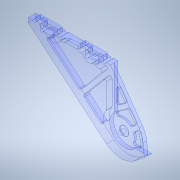
# Autodesk Inventor part: 後ろウィング固定フレームver2(ミラー)反対側
Saved by Autodesk Inventor 2020.2 (Build 242310000, 310)
## iProperties
Created: 2020-05-07
Part Number: 後ろウィング固定フレームver2(ミラー)反対側
Material: ポリカーボネート、クリア
Document SubType Name: Modeling
Designer: mozar
Density: 1.2 g/cm^3
Appearance: ポリカーボネート - クリア
Mass: 7.61117 g
Surface Area: 65.4566 cm^2
Volume: 6.34264 cm^3
Author: mozar
Autodesk Inventor part; units mm, degrees
(part 1 of 2)
ref_plane "YZ Plane" through (0, 0, 0) normal (1, 0, 0) x (0, 1, 0)
ref_plane "XZ Plane" through (0, 0, 0) normal (0, 1, 0) x (-1, 0, 0)
ref_plane "XY Plane" through (0, 0, 0) normal (0, 0, 1) x (1, 0, 0)
sketch "スケッチ1" plane through (0, 0, 0) normal (0, 0, 1) x (1, 0, 0)
  line L0 (-101.5, 47.999998) -> (108.5, 47.999998)
  circle A0 centre (111.885049, -39.000002) radius 4
  circle A1 centre (191.876682, -37.842982) radius 4
  circle A2 centre (111.885049, -39.000002) radius 7
  circle A3 centre (191.876682, -37.842982) radius 7
  line L1 (191.876682, -37.842982) -> (111.885049, -39.000002) construction
  line L2 (191.775442, -30.843714) -> (111.78381, -32.000734)
  line L3 (111.986288, -45.99927) -> (191.977921, -44.84225)
  arc A4 (191.977921, -44.84225) -> (191.775442, -30.843714) centre (191.876682, -37.842982) ccw
  arc A5 (111.78381, -32.000734) -> (111.986288, -45.99927) centre (111.885049, -39.000002) ccw
  line L4 (193.542302, -31.044032) -> (241.704818, -42.842982)
  circle A6 centre (234.566446, -71.981335) radius 30
  line L5 (262.587356, -82.697145) -> (213.725294, -50.402494)
  line L6 (213.725294, -50.402494) -> (190.211062, -44.641931)
  line L7 (264.566446, -121.542906) -> (264.566446, -63.2267)
  line L8 (111.885049, -39.000002) -> (111.885049, 40.999998) construction
  line L9 (118.885049, -39.000002) -> (118.885049, 40.999998)
  line L10 (104.885049, 40.999998) -> (104.885049, -39.000002)
  arc A7 (104.885049, -39.000002) -> (118.885049, -39.000002) centre (111.885049, -39.000002) ccw
  arc A8 (118.885049, 40.999998) -> (104.885049, 40.999998) centre (111.885049, 40.999998) ccw
  circle A9 centre (58.238326, 51.481995) radius 30
  line L11 (113.558078, 34.202868) -> (65.408448, 22.351438)
  line L12 (28.441083, 47.999998) -> (86.70408, 42.010942)
  line L13 (86.70408, 42.010942) -> (110.21202, 47.797128)
  circle A10 centre (113.5, -20.000002) radius 68
  line L14 (315.327237, -100.585467) -> (70.600424, 104.764712)
  line L15 (253.850074, -49.000002) -> (111.885049, -39.000002)
  arc A11 (93.592427, -27.104845) -> (135.370976, -5.924402) centre (95.060351, 21.794105) ccw
  arc A12 (135.370976, -5.924402) -> (135.847591, -3.671647) centre (132.898992, -4.224609) ccw
  arc A13 (135.847591, -3.671647) -> (83.183341, 18.55647) centre (102.157897, -9.989602) ccw
  line L16 (111.885049, -39.000002) -> (112.74718, 40.995353) construction
  line L17 (118.884642, -39.075438) -> (119.746773, 40.919916)
  line L18 (105.747586, 41.070789) -> (104.885455, -38.924565)
  arc A14 (104.885455, -38.924565) -> (118.884642, -39.075438) centre (111.885049, -39.000002) ccw
  arc A15 (119.746773, 40.919916) -> (105.747586, 41.070789) centre (112.74718, 40.995353) ccw
  line L19 (164.994898, 47.999998) -> (164.994898, 25.999998)
  line L20 (164.994898, 25.999998) -> (327.494898, -102.000002)
  circle A16 centre (116.292557, -40.000002) radius 68
  circle A17 centre (-98.885049, -0.000002) radius 67.5
  line L21 (321.363327, -8.500986) -> (-152.668056, 78.49822)
  line L22 (104.889695, -3) -> (104.889695, 0)
  line L23 (104.889695, -3) -> (64.444342, -3)
  line L24 (72.06562, 0) -> (104.889695, 0)
  circle A18 centre (83.376901, -17.5) radius 13.85
  line L25 (198.510163, -35.607602) -> (190.779082, -12.66564)
  line L26 (185.2432, -40.078361) -> (169.408182, 6.912014)
  circle A19 centre (197.837389, 16.492211) radius 30
  line L27 (190.779082, -12.66564) -> (191.876682, 45.894081)
  circle A20 centre (191.876682, -37.842982) radius 83.737063
  line L28 (191.876682, 45.894081) -> (191.876682, -37.842982)
  line L29 (96.889695, -3) -> (96.889695, -6)
  line L30 (96.889695, -6) -> (87.889695, -6)
  line L31 (87.889695, -6) -> (87.889695, -3)
  line L32 (76.444342, -3) -> (76.444342, -6)
  line L33 (76.444342, -6) -> (67.444342, -6)
  line L34 (67.444342, -6) -> (67.444342, -3)
  line L35 (99.889695, -3) -> (99.889695, 0)
  line L36 (99.889695, 0) -> (84.889695, 0)
  line L37 (84.889695, 0) -> (84.889695, -3)
  line L38 (79.444342, -3) -> (79.444342, 0)
  line L39 (79.444342, 0) -> (64.444342, 0)
  line L40 (64.444342, 0) -> (64.444342, -3)
  line L41 (64.444342, 0) -> (59.444342, 0)
  line L42 (59.444342, 0) -> (59.444342, -3)
  line L43 (59.444342, -3) -> (64.444342, -3)
  line L44 (59.444342, -3) -> (59.444342, -6)
  circle A21 centre (111.885049, -39.000002) radius 1.5
  circle A22 centre (111.885049, -39.000002) radius 9
  circle A23 centre (111.885049, -39.000002) radius 10
  circle A24 centre (111.885049, -39.000002) radius 15
  line L45 (121.057661, -50.868582) -> (142.927269, -50.552254)
  line L46 (121.057661, -50.868582) -> (127.651316, -45.772687)
  line L47 (127.651316, -45.772687) -> (126.808053, -37.482129)
  line L48 (124.15135, -30.366471) -> (104.889695, -3)
  line L49 (101.060181, -49.383751) -> (59.444342, -6)
  circle A25 centre (95.889695, -6) radius 1
  circle A26 centre (88.889695, -6) radius 1
  circle A27 centre (95.889695, -3) radius 1
  circle A28 centre (88.889695, -3) radius 1
  circle A29 centre (100.889695, -3) radius 1
  circle A30 centre (83.889695, -3) radius 1
  circle A31 centre (80.444342, -3) radius 1
  circle A32 centre (75.444342, -6) radius 1
  circle A33 centre (68.444342, -6) radius 1
  circle A34 centre (75.444342, -3) radius 1
  circle A35 centre (68.444342, -3) radius 1
  circle A36 centre (63.444342, -3) radius 1
  point P0 (0, 0)
  point P1 (151.880865, -38.421492)
  point P2 (111.885049, 0.999998)
  point P3 (105.885049, -0.000002)
  point P4 (105.885049, -0.000002)
  point P5 (23.732778, -42.728965)
  point P6 (112.316114, 0.997675)
  point P7 (99.889695, -1.5)
  point P8 (76.444342, -4.5)
  point P9 (74.444342, -6)
  point P10 (69.444342, -6)
  point P11 (69.444342, -3)
  point P12 (74.444342, -3)
  point P13 (82.889695, -3)
  point P14 (81.444342, -3)
  point P15 (62.444342, -3)
  point P16 (101.889695, -3)
  point P17 (89.889695, -3)
  point P18 (94.889695, -3)
  point P19 (94.889695, -6)
  point P20 (89.889695, -6)
  point P21 (118.961603, -31.934425)
  point P22 (118.924491, -31.897449)
  point P23 (118.962007, -31.896907)
  point P24 (119.12697, -45.895985)
  point P25 (104.885049, -3)
  point P26 (104.885049, -31.858573)
  dimension "d27" = 167.47413
  dimension "d0" = 8
  dimension "d1" = 8
  dimension "d2" = 3
  dimension "d3" = 3
  dimension "d4" = 80
  dimension "d5" = 14
  dimension "d6" = 14
  dimension "d7" = 60
  dimension "d8" = 14
  dimension "d9" = 60
  dimension "d10" = 14
  dimension "d11" = 6
  dimension "d12" = 40
  dimension "d13" = 13.271
  dimension "d14" = 14
  dimension "d15" = 10
  dimension "d16" = 5
  dimension "d17" = 22
  dimension "d18" = 150
  dimension "d19" = 162.5
  dimension "d20" = 0
  dimension "d21" = 136
  dimension "d22" = 136
  dimension "d23" = 135
  dimension "d24" = 38.2272
  dimension "d25" = 25
  dimension "d26" = 60
  dimension "d28" = 5
  dimension "d29" = 3
  dimension "d30" = 5
  dimension "d31" = 3
  dimension "d32" = 3
  dimension "d33" = 5
  dimension "d34" = 1
  dimension "d35" = 5
  dimension "d36" = 5
  dimension "d37" = 2
  dimension "d38" = 2
  dimension "d39" = 2
  dimension "d40" = 2
  dimension "d41" = 2
  dimension "d42" = 2
  dimension "d43" = 2
  dimension "d44" = 2
  dimension "d45" = 2
  dimension "d46" = 2
  dimension "d47" = 2
  dimension "d48" = 2
  constraints: 104 end point, 46 tangent, 37 point on circle, 36 centre point, 14 vertical, 8 point on line, 7 equal length, 7 horizontal, 5 coincident, 5 midpoint, 5 parallel, 1 concentric, 1 perpendicular, 1 vertical alignment, 25 other
  measures "d0" diameter of A0
  measures "d1" diameter of A1
  measures "d2" radial gap between concentric circles of A0 A2
  measures "d3" radial gap between concentric circles of A1 A3
  measures "d4" distance of L1.start L1.end
  measures "d5" diameter of A5
  measures "d6" distance from line of L4 L5.end
  measures "d7" diameter of A6
  measures "d8" diameter of A8
  measures "d9" diameter of A9
  measures "d10" distance from line of L11 L12.end
  measures "d11" horizontal distance of L1.end point (105.885, 0)
  measures "d12" angle of L14 L0
  measures "d14" diameter of A15
  measures "d15" vertical distance of L15.start L1.end
  measures "d16" vertical distance of L1.start L4.end
  measures "d17" distance of L19.start L19.end
  measures "d18" vertical distance of L19.start L20.end
  measures "d19" distance from line of L19 L20.end
  measures "d20" distance from line of L19.start L0
  measures "d21" diameter of A10
  measures "d22" diameter of A16
  measures "d23" diameter of A17
  measures "d24" angle of L0 L20
  measures "d25" distance from line of L5.start L20
  measures "d26" diameter of A19
  measures "d28" distance between parallel lines of L35 L22
  measures "d29" distance of L41.end L42.end
  measures "d30" distance of L42.end L40.end
  measures "d31" distance of L42.end L44.end
  measures "d32" diameter of A21
  measures "d33" radial gap between concentric circles of A0 A22
  measures "d34" radial gap between concentric circles of A22 A23
  measures "d35" radial gap between concentric circles of A23 A24
  measures "d36" distance between parallel lines of L3 L45
  measures "d37" diameter of A25
  measures "d38" diameter of A26
  measures "d39" diameter of A27
  measures "d40" diameter of A28
  measures "d41" diameter of A29
  measures "d42" diameter of A30
  measures "d43" diameter of A31
  measures "d44" diameter of A32
  measures "d45" diameter of A33
  measures "d46" diameter of A34
  measures "d47" diameter of A35
  measures "d48" diameter of A36
extrude "押し出し1" add sketch "スケッチ1" against normal blind 5 contours A24 A11 L10 A23 A20 | A20 A23 L3 A24 | L43 A36 L23 L34 A33 L33 A32 A18 L49 L44 | L46 A24 L3 | L3 A24 L15 L47 | A23 L10 A22 A20 | A20 A22 L3 A23 | L49 A18 L30 A25 L29 L23 A29 L10 A24 | L39 L24 L38 L23 A34 A35 L40 | L3 A23 L15 A24 | L15 A24 L47 | A22 L10 A2 A20 | A20 A2 L3 A22 | A23 L18 A22 L10 | L10 A11 L18 A23 | L3 A22 L15 A23 | A24 L10 A11 | L49 A18 A32 L32 A31 A30 L31 A26 L30 | L15 A23 L17 L2 A24 | L2 L17 A24 | A20 A0 L15 A2 | A2 A20 A0 | A22 L18 L10 | L3 A2 L15 A22 | L10 A24 L18 A11 | A23 A20 A22 L18 | L18 A11 A20 A23 | L15 A22 L17 A23 | L10 L23 L48 L18 A24 | L35 L23 A27 A28 L37 L24 | L48 A20 A24 L18 | L17 A23 L2 | L2 A23 L9 A24 L17 | A24 L17 L48 | A20 A0 | A0 A20 | L18 A22 A20 A2 | L15 A2 L17 A22 | L18 A24 A20 A11 | A23 L9 L2 A22 A20 | A20 A11 A24 L9 A23 | A31 A18 L32 L23 | L48 A11 A24 A20 | A23 L17 A22 L9 L2 | L2 L9 A23 | A24 L9 L48 L17 | L15 A0 A20 A2 | A20 A22 L2 A2 | A20 A24 A11 | A18 A30 L23 L31 | L23 A30 A18 A31 | L48 L9 A24 A11 | L9 A22 L2 | L17 L9 A22 | L2 A22 L9 A2
extrude "押し出し2" cut sketch "スケッチ1" against normal blind 2.55 contours L3 A24 L15 L47 | A23 L10 A22 A20 | A20 A22 L3 A23 | L3 A23 L15 A24 | L15 A24 L47 | A22 L10 A2 A20 | A20 A2 L3 A22 | A23 L18 A22 L10 | L10 A11 L18 A23 | L3 A22 L15 A23 | L15 A23 L17 L2 A24 | L2 L17 A24 | A20 A0 L15 A2 | A2 A20 A0 | A22 L18 L10 | L3 A2 L15 A22 | L10 A24 L18 A11 | A23 A20 A22 L18 | L18 A11 A20 A23 | L15 A22 L17 A23 | L10 L23 L48 L18 A24 | L48 A20 A24 L18 | L17 A23 L2 | L2 A23 L9 A24 L17 | A24 L17 L48 | A20 A0 | A0 A20 | L18 A22 A20 A2 | L15 A2 L17 A22 | L18 A24 A20 A11 | A23 L9 L2 A22 A20 | A20 A11 A24 L9 A23 | L48 A11 A24 A20 | A23 L17 A22 L9 L2 | L2 L9 A23 | A24 L9 L48 L17 | L15 A0 A20 A2 | A20 A22 L2 A2 | A20 A24 A11 | L48 L9 A24 A11 | L9 A22 L2 | L17 L9 A22 | L2 A22 L9 A2 | A21
sketch "スケッチ2" plane through (0, 0, 0) normal (0, 0, 1) x (1, 0, 0)
  line L0 (87.889695, -6) -> (87.889695, -3)
  arc A0 (89.889695, -3) -> (87.889695, -3) centre (88.889695, -3) ccw
  line L1 (89.889695, -3) -> (94.889695, -3)
  arc A1 (96.889695, -3) -> (94.889695, -3) centre (95.889695, -3) ccw
  line L2 (96.889695, -3) -> (96.889695, -6)
  arc A2 (94.889695, -6) -> (96.889695, -6) centre (95.889695, -6) ccw
  line L3 (94.889695, -6) -> (89.889695, -6)
  arc A3 (87.889695, -6) -> (89.889695, -6) centre (88.889695, -6) ccw
  arc A4 (67.444342, -6) -> (69.444342, -6) centre (68.444342, -6) ccw
  line L4 (67.444342, -6) -> (67.444342, -3)
  arc A5 (69.444342, -3) -> (67.444342, -3) centre (68.444342, -3) ccw
  line L5 (69.444342, -3) -> (74.444342, -3)
  arc A6 (76.444342, -3) -> (74.444342, -3) centre (75.444342, -3) ccw
  line L6 (76.444342, -3) -> (76.444342, -6)
  arc A7 (74.444342, -6) -> (76.444342, -6) centre (75.444342, -6) ccw
  line L7 (74.444342, -6) -> (69.444342, -6)
  line L8 (127.651316, -45.772687) -> (119.12697, -45.895985)
  arc A8 (104.885049, -31.858573) -> (119.12697, -45.895985) centre (111.885049, -39.000002) ccw
  line L9 (104.885049, -31.858573) -> (104.885049, -3)
  line L10 (104.885049, -3) -> (101.889695, -3)
  arc A9 (99.889695, -3) -> (101.889695, -3) centre (100.889695, -3) ccw
  line L11 (99.889695, -3) -> (99.889695, 0)
  line L12 (99.889695, 0) -> (84.889695, 0)
  line L13 (84.889695, 0) -> (84.889695, -3)
  arc A10 (82.889695, -3) -> (84.889695, -3) centre (83.889695, -3) ccw
  line L14 (82.889695, -3) -> (81.444342, -3)
  arc A11 (79.444342, -3) -> (81.444342, -3) centre (80.444342, -3) ccw
  line L15 (79.444342, -3) -> (79.444342, 0)
  line L16 (79.444342, 0) -> (64.444342, 0)
  line L17 (64.444342, 0) -> (64.444342, -3)
  arc A12 (62.444342, -3) -> (64.444342, -3) centre (63.444342, -3) ccw
  line L18 (62.444342, -3) -> (59.444342, -3)
  line L19 (59.444342, -3) -> (59.444342, -6)
  line L20 (59.444342, -6) -> (101.060181, -49.383751)
  arc A13 (101.060181, -49.383751) -> (121.057661, -50.868582) centre (111.885049, -39.000002) ccw
  line L21 (121.057661, -50.868582) -> (127.651316, -45.772687)
  circle A14 centre (111.885049, -39.000002) radius 1.5
  circle A15 centre (111.885049, -39.000002) radius 3
  point P0 (0, 0)
  dimension "d53" = 6
  constraints: 1 centre point, 1 coincident
  measures "d53" diameter of A15
extrude "押し出し3" cut sketch "スケッチ2" against normal blind 3 contours A15
sketch "スケッチ3" plane through (0, 0, 0) normal (0, 0, 1) x (1, 0, 0)
  line L0 (87.889695, -6) -> (87.889695, -3)
  arc A0 (89.889695, -3) -> (87.889695, -3) centre (88.889695, -3) ccw
  line L1 (89.889695, -3) -> (94.889695, -3)
  arc A1 (96.889695, -3) -> (94.889695, -3) centre (95.889695, -3) ccw
  line L2 (96.889695, -3) -> (96.889695, -6)
  arc A2 (94.889695, -6) -> (96.889695, -6) centre (95.889695, -6) ccw
  line L3 (94.889695, -6) -> (89.889695, -6)
  arc A3 (87.889695, -6) -> (89.889695, -6) centre (88.889695, -6) ccw
  arc A4 (67.444342, -6) -> (69.444342, -6) centre (68.444342, -6) ccw
  line L4 (67.444342, -6) -> (67.444342, -3)
  arc A5 (69.444342, -3) -> (67.444342, -3) centre (68.444342, -3) ccw
  line L5 (69.444342, -3) -> (74.444342, -3)
  arc A6 (76.444342, -3) -> (74.444342, -3) centre (75.444342, -3) ccw
  line L6 (76.444342, -3) -> (76.444342, -6)
  arc A7 (74.444342, -6) -> (76.444342, -6) centre (75.444342, -6) ccw
  line L7 (74.444342, -6) -> (69.444342, -6)
  line L8 (127.651316, -45.772687) -> (119.12697, -45.895985)
  arc A8 (104.885049, -31.858573) -> (119.12697, -45.895985) centre (111.885049, -39.000002) ccw
  line L9 (104.885049, -31.858573) -> (104.885049, -3)
  line L10 (104.885049, -3) -> (101.889695, -3)
  arc A9 (99.889695, -3) -> (101.889695, -3) centre (100.889695, -3) ccw
  line L11 (99.889695, -3) -> (99.889695, 0)
  line L12 (99.889695, 0) -> (84.889695, 0)
  line L13 (84.889695, 0) -> (84.889695, -3)
  arc A10 (82.889695, -3) -> (84.889695, -3) centre (83.889695, -3) ccw
  line L14 (82.889695, -3) -> (81.444342, -3)
  arc A11 (79.444342, -3) -> (81.444342, -3) centre (80.444342, -3) ccw
  line L15 (79.444342, -3) -> (79.444342, 0)
  line L16 (79.444342, 0) -> (64.444342, 0)
  line L17 (64.444342, 0) -> (64.444342, -3)
  arc A12 (62.444342, -3) -> (64.444342, -3) centre (63.444342, -3) ccw
  line L18 (62.444342, -3) -> (59.444342, -3)
  line L19 (59.444342, -3) -> (59.444342, -6)
  line L20 (59.444342, -6) -> (101.060181, -49.383751)
  arc A13 (101.060181, -49.383751) -> (121.057661, -50.868582) centre (111.885049, -39.000002) ccw
  line L21 (121.057661, -50.868582) -> (127.651316, -45.772687)
  line L22 (99.889695, 0) -> (99.889695, -3)
  line L23 (99.889695, 0) -> (64.444342, 0)
  line L24 (64.444342, 0) -> (64.444342, -3)
  line L25 (64.444342, -3) -> (99.889695, -3)
  line L26 (99.889695, -3) -> (99.889695, 0)
  point P0 (0, 0)
  constraints: 8 end point, 2 parallel, 1 horizontal, 1 perpendicular
extrude "押し出し4" cut sketch "スケッチ3" against normal blind 2 contours L25 L13 L12 L11 A1 L1 A0 | A0 L25 | L25 L14 L15 L23 L13 | A1 L25 | L15 L25 A6 L5 A5 L17 L16 | L25 A6 | A5 L25
sketch "スケッチ4" plane through (0, 0, -5) normal (0, 0, -1) x (-1, 0, 0)
  circle A0 centre (-111.885049, -39.000002) radius 3
  line L0 (-104.885049, -3) -> (-104.889695, -3)
  line L1 (-104.885049, -31.858573) -> (-104.885049, -3)
  arc A1 (-119.12697, -45.895985) -> (-104.885049, -31.858573) centre (-111.885049, -39.000002) ccw
  line L2 (-127.651316, -45.772687) -> (-119.12697, -45.895985)
  line L3 (-126.808053, -37.482129) -> (-127.651316, -45.772687)
  arc A2 (-124.15135, -30.366471) -> (-126.808053, -37.482129) centre (-111.885049, -39.000002) ccw
  line L4 (-104.889695, -3) -> (-124.15135, -30.366471)
  circle A3 centre (-111.885049, -39.000002) radius 1.5
  point P0 (0, 0)
sketch "スケッチ5" plane through (0, 0, 0) normal (0, 0, 1) x (1, 0, 0)
  circle A0 centre (111.885049, -39.000002) radius 3
  line L0 (104.885049, -3) -> (104.889695, -3)
  line L1 (104.885049, -31.858573) -> (104.885049, -3)
  arc A1 (104.885049, -31.858573) -> (119.12697, -45.895985) centre (111.885049, -39.000002) ccw
  line L2 (127.651316, -45.772687) -> (119.12697, -45.895985)
  line L3 (126.808053, -37.482129) -> (127.651316, -45.772687)
  arc A2 (126.808053, -37.482129) -> (124.15135, -30.366471) centre (111.885049, -39.000002) ccw
  line L4 (104.889695, -3) -> (124.15135, -30.366471)
  circle A3 centre (111.885049, -39.000002) radius 1.5
  point P0 (0, 0)
extrude "押し出し5" add sketch "スケッチ5" against normal blind 3 contours A0 | L0 L4 A2 L3 L2 A1 L1
extrude "押し出し6" cut sketch "スケッチ4" against normal blind 3 contours A0
extrude "押し出し7" cut sketch "スケッチ4" against normal blind 2.55 contours L1 A1 L2 L3 A2 L4 L0
sketch "スケッチ6" plane through (0, 0, -5) normal (0, 0, -1) x (-1, 0, 0)
  line L0 (-79.444342, 0) -> (-79.444342, -3)
  line L1 (-64.444342, 0) -> (-79.444342, 0)
  line L2 (-64.444342, -3) -> (-64.444342, 0)
  line L3 (-67.444342, -3) -> (-64.444342, -3)
  arc A0 (-67.444342, -3) -> (-69.444342, -3) centre (-68.444342, -3) ccw
  line L4 (-74.444342, -3) -> (-69.444342, -3)
  arc A1 (-74.444342, -3) -> (-76.444342, -3) centre (-75.444342, -3) ccw
  line L5 (-79.444342, -3) -> (-76.444342, -3)
  arc A2 (-94.889695, -3) -> (-96.889695, -3) centre (-95.889695, -3) ccw
  line L6 (-99.889695, -3) -> (-96.889695, -3)
  line L7 (-99.889695, 0) -> (-99.889695, -3)
  line L8 (-84.889695, 0) -> (-99.889695, 0)
  line L9 (-84.889695, -3) -> (-84.889695, 0)
  line L10 (-87.889695, -3) -> (-84.889695, -3)
  arc A3 (-87.889695, -3) -> (-89.889695, -3) centre (-88.889695, -3) ccw
  line L11 (-94.889695, -3) -> (-89.889695, -3)
  point P0 (0, 0)
sketch "スケッチ7" plane through (0, 0, 0) normal (0, 0, 1) x (1, 0, 0)
  arc A0 (96.889695, -3) -> (94.889695, -3) centre (95.889695, -3) ccw
  line L0 (99.889695, -3) -> (96.889695, -3)
  line L1 (99.889695, 0) -> (99.889695, -3)
  line L2 (84.889695, 0) -> (99.889695, 0)
  line L3 (84.889695, -3) -> (84.889695, 0)
  line L4 (87.889695, -3) -> (84.889695, -3)
  arc A1 (89.889695, -3) -> (87.889695, -3) centre (88.889695, -3) ccw
  line L5 (94.889695, -3) -> (89.889695, -3)
  line L6 (79.444342, 0) -> (79.444342, -3)
  line L7 (64.444342, 0) -> (79.444342, 0)
  line L8 (64.444342, -3) -> (64.444342, 0)
  line L9 (67.444342, -3) -> (64.444342, -3)
  arc A2 (69.444342, -3) -> (67.444342, -3) centre (68.444342, -3) ccw
  line L10 (74.444342, -3) -> (69.444342, -3)
  arc A3 (76.444342, -3) -> (74.444342, -3) centre (75.444342, -3) ccw
  line L11 (79.444342, -3) -> (76.444342, -3)
  point P0 (0, 0)
extrude "押し出し8" add sketch "スケッチ7" against normal blind 5
extrude "押し出し9" cut sketch "スケッチ6" against normal blind 2
sketch "スケッチ8" plane through (0, 0, -5) normal (0, 0, -1) x (-1, 0, 0)
  line L0 (-84.889695, -3) -> (-87.889695, -3)
  line L1 (-87.889695, -3) -> (-87.889695, -6)
  arc A0 (-89.889695, -6) -> (-87.889695, -6) centre (-88.889695, -6) ccw
  line L2 (-89.889695, -6) -> (-94.889695, -6)
  arc A1 (-96.889695, -6) -> (-94.889695, -6) centre (-95.889695, -6) ccw
  line L3 (-96.889695, -6) -> (-96.889695, -3)
  line L4 (-96.889695, -3) -> (-99.889695, -3)
  arc A2 (-101.889695, -3) -> (-99.889695, -3) centre (-100.889695, -3) ccw
  line L5 (-101.889695, -3) -> (-104.885049, -3)
  line L6 (-104.885049, -3) -> (-104.885049, -31.858573)
  arc A3 (-119.12697, -45.895985) -> (-104.885049, -31.858573) centre (-111.885049, -39.000002) ccw
  line L7 (-119.12697, -45.895985) -> (-127.651316, -45.772687)
  line L8 (-127.651316, -45.772687) -> (-121.057661, -50.868582)
  arc A4 (-121.057661, -50.868582) -> (-101.060181, -49.383751) centre (-111.885049, -39.000002) ccw
  line L9 (-101.060181, -49.383751) -> (-59.444342, -6)
  line L10 (-59.444342, -6) -> (-59.444342, -3)
  line L11 (-59.444342, -3) -> (-62.444342, -3)
  arc A5 (-64.444342, -3) -> (-62.444342, -3) centre (-63.444342, -3) ccw
  line L12 (-64.444342, -3) -> (-67.444342, -3)
  line L13 (-67.444342, -3) -> (-67.444342, -6)
  arc A6 (-69.444342, -6) -> (-67.444342, -6) centre (-68.444342, -6) ccw
  line L14 (-69.444342, -6) -> (-74.444342, -6)
  arc A7 (-76.444342, -6) -> (-74.444342, -6) centre (-75.444342, -6) ccw
  line L15 (-76.444342, -6) -> (-76.444342, -3)
  line L16 (-76.444342, -3) -> (-79.444342, -3)
  arc A8 (-81.444342, -3) -> (-79.444342, -3) centre (-80.444342, -3) ccw
  line L17 (-81.444342, -3) -> (-82.889695, -3)
  arc A9 (-84.889695, -3) -> (-82.889695, -3) centre (-83.889695, -3) ccw
  line L18 (-66.444342, -6) -> (-57.444342, -6)
  line L19 (-57.444342, -6) -> (-57.444342, -3)
  line L20 (-57.444342, -3) -> (-66.444342, -3)
  line L21 (-66.444342, -3) -> (-66.444342, -6)
  line L22 (-69.444342, -6) -> (-74.444342, -6)
  line L23 (-64.444342, -3) -> (-67.444342, -3)
  circle A10 centre (-65.444342, -3) radius 1
  circle A11 centre (-65.444342, -6) radius 1
  circle A12 centre (-58.444342, -3) radius 1
  circle A13 centre (-58.444342, -6) radius 1
  line L24 (-54.444342, 0) -> (-54.444342, -6)
  line L25 (-61.090093, -9) -> (-62.79859, -9)
  line L26 (-69.444342, -6) -> (-69.444342, 0)
  line L27 (-69.444342, 0) -> (-54.444342, 0)
  circle A14 centre (-65.444342, -6) radius 4
  circle A15 centre (-58.444342, -6) radius 4
  line L28 (-64.444342, 0) -> (-64.444342, -3)
  line L29 (-79.444342, -3) -> (-79.444342, 0)
  line L30 (-69.444342, 0) -> (-54.444342, 0)
  line L31 (-54.444342, 0) -> (-54.444342, -3)
  line L32 (-54.444342, -3) -> (-69.444342, -3)
  line L33 (-69.444342, -3) -> (-69.444342, 0)
  line L34 (-54.444342, -3) -> (-49.444342, -3)
  line L35 (-49.444342, -3) -> (-49.444342, -6)
  line L36 (-49.444342, -6) -> (-54.444342, -6)
  line L37 (-54.444342, -6) -> (-54.444342, -3)
  circle A16 centre (-53.444342, -3) radius 1
  circle A17 centre (-70.444342, -3) radius 1
  line L38 (-76.444342, -3) -> (-69.444342, -3)
  line L39 (-79.444342, 0) -> (-64.444342, 0)
  line L40 (-79.444342, 0) -> (-64.444342, 0)
  line L41 (-81.444342, -3) -> (-79.444342, -3)
  point P0 (0, 0)
  point P1 (-61.944342, -3)
  point P2 (-52.444342, -3)
  point P3 (-71.444342, -3)
  point P4 (-59.444342, -6)
  point P5 (-64.444342, -6)
  dimension "d68" = 9
  dimension "d69" = 3
  dimension "d70" = 10
  dimension "d71" = 2
  dimension "d72" = 2
  dimension "d73" = 2
  dimension "d74" = 2
  dimension "d75" = 3
  dimension "d76" = 3
  dimension "d77" = 3
  dimension "d78" = 3
  dimension "d79" = 15
  dimension "d80" = 15
  dimension "d81" = 3
  dimension "d82" = 3
  dimension "d83" = 15
  dimension "d84" = 3
  dimension "d85" = 10
  dimension "d86" = 2
  dimension "d88" = 2
  constraints: 38 end point, 8 centre point, 8 parallel, 7 point on line, 7 tangent, 4 horizontal, 4 perpendicular, 4 point on circle, 2 midpoint, 1 collinear
  measures "d68" distance of L20.end L19.end
  measures "d69" distance of L19.end L18.end
  measures "d70" distance between parallel lines of L15 L21
  measures "d71" diameter of A10
  measures "d72" diameter of A11
  measures "d73" diameter of A12
  measures "d74" diameter of A13
  measures "d75" distance between parallel lines of L19 L24
  measures "d76" radial gap between concentric circles of A11 A14
  measures "d77" radial gap between concentric circles of A13 A15
  measures "d78" distance between parallel lines of L14 L25
  measures "d79" distance between parallel lines of L28 L29
  measures "d80" distance of L31.end L32.end
  measures "d81" distance of L30.end L31.end
  measures "d82" distance between parallel lines of L32 L27
  measures "d83" distance between parallel lines of L31 L33
  measures "d84" distance of L34.end L35.end
  measures "d85" distance between parallel lines of L35 L10
  measures "d86" diameter of A16
  measures "d88" diameter of A17
extrude "押し出し10" cut sketch "スケッチ8" against normal blind 10 contours L29 L39 L26 A17 L38 L16 | A17 L38 | L27 L28 A14 L32 L26 | A14 A10 L12 L32 | L28 A10 A14 | A10 L12 picked at (-70.194838, -2.619415) picked at (-65.236512, -2.450134)
extrude "押し出し11" add sketch "スケッチ8" against normal blind 5 contours L38 A17 L26 L14 A7 L15 | L27 L28 A14 L32 L26 | L32 A14 L26 | L27 L24 L32 A15 L11 L20 A14 L28 | A14 L32 L13 A6 | A6 L13 L12 L21 A11 L18 A15 A14 | A14 A10 L12 L32 | L28 A10 A14 | A14 L20 L28 | A14 A15 L9 L25 | A10 L12 | A16 L34 L35 L36 L24 | L24 A15 L32 | A14 A5 L20 | L20 A5 A14 | A10 L12 | A5 A14 A15 L18 A11 L21 A10 | L9 A15 L25 | A15 L18 A14 | A14 L18 L9 A15 | A15 L9 A13 L19 L32 | L32 A12 A15 | L11 A15 A14 A5 | A14 A15 L11 L10 L18 | L18 A15 A14 | A12 L20 | A12 L11 A15 | A12 L20 | L19 A13 L10 A12 | A13 L18 | L18 A13
extrude "押し出し12" cut sketch "スケッチ8" against normal blind 10 contours A10 L12 | A14 A5 L20 | L20 A5 A14 | A10 L12 | A5 A14 A15 L18 A11 L21 A10 | L11 A15 A14 A5 | A14 A15 L11 L10 L18 | L18 A15 A14 | A11 L18 | L18 A11 | A12 L20 | A12 L20 | L19 A13 L10 A12 | A13 L18 | L18 A13 picked at (-61.796548, -5.776456)
extrude "押し出し13" add sketch "スケッチ8" against normal blind 5 contours L41 A8
sketch "スケッチ9" plane through (0, 0, -5) normal (0, 0, -1) x (-1, 0, 0)
  line L0 (-59.444342, -6) -> (-64.444342, -6)
  arc A0 (-66.444342, -6) -> (-64.444342, -6) centre (-65.444342, -6) ccw
  line L1 (-66.444342, -6) -> (-66.444342, -3)
  arc A1 (-64.444342, -3) -> (-66.444342, -3) centre (-65.444342, -3) ccw
  line L2 (-64.444342, -3) -> (-59.444342, -3)
  arc A2 (-57.444342, -3) -> (-59.444342, -3) centre (-58.444342, -3) ccw
  line L3 (-57.444342, -3) -> (-57.444342, -6)
  arc A3 (-59.444342, -6) -> (-57.444342, -6) centre (-58.444342, -6) ccw
  line L4 (-62.32209, -9) -> (-61.090093, -9)
  arc A4 (-61.090093, -9) -> (-54.444342, -6) centre (-58.444342, -6) ccw
  line L5 (-54.444342, -6) -> (-49.444342, -6)
  line L6 (-49.444342, -6) -> (-49.444342, -3)
  line L7 (-49.444342, -3) -> (-52.444342, -3)
  arc A5 (-54.444342, -3) -> (-52.444342, -3) centre (-53.444342, -3) ccw
  line L8 (-54.444342, -3) -> (-54.444342, 0)
  line L9 (-54.444342, 0) -> (-69.444342, 0)
  line L10 (-69.444342, 0) -> (-69.444342, -3)
  arc A6 (-71.444342, -3) -> (-69.444342, -3) centre (-70.444342, -3) ccw
  line L11 (-71.444342, -3) -> (-82.889695, -3)
  arc A7 (-84.889695, -3) -> (-82.889695, -3) centre (-83.889695, -3) ccw
  line L12 (-84.889695, -3) -> (-87.889695, -3)
  line L13 (-87.889695, -3) -> (-87.889695, -6)
  arc A8 (-89.889695, -6) -> (-87.889695, -6) centre (-88.889695, -6) ccw
  line L14 (-89.889695, -6) -> (-94.889695, -6)
  arc A9 (-96.889695, -6) -> (-94.889695, -6) centre (-95.889695, -6) ccw
  line L15 (-96.889695, -6) -> (-96.889695, -3)
  line L16 (-96.889695, -3) -> (-99.889695, -3)
  arc A10 (-101.889695, -3) -> (-99.889695, -3) centre (-100.889695, -3) ccw
  line L17 (-101.889695, -3) -> (-104.885049, -3)
  line L18 (-104.885049, -3) -> (-104.885049, -31.858573)
  arc A11 (-119.12697, -45.895985) -> (-104.885049, -31.858573) centre (-111.885049, -39.000002) ccw
  line L19 (-119.12697, -45.895985) -> (-127.651316, -45.772687)
  line L20 (-127.651316, -45.772687) -> (-121.057661, -50.868582)
  arc A12 (-121.057661, -50.868582) -> (-101.060181, -49.383751) centre (-111.885049, -39.000002) ccw
  line L21 (-101.060181, -49.383751) -> (-62.32209, -9)
  circle A13 centre (-111.885049, -39.000002) radius 1.5
  line L22 (-101.060181, -49.383751) -> (-62.32209, -9)
  circle A14 centre (-111.885049, -39.000002) radius 15
  line L23 (-54.444342, -6) -> (-49.444342, -6)
  arc A15 (-121.057661, -50.868582) -> (-101.060181, -49.383751) centre (-111.885049, -39.000002) ccw
  line L24 (-102.219392, -50.47062) -> (-49.444342, -6)
  point P0 (0, 0)
  constraints: 2 end point, 1 coincident, 1 point on circle, 4 other
extrude "押し出し14" add sketch "スケッチ9" against normal blind 5 contours L4 A4 L5 L24 A12 L21
extrude "押し出し15" cut sketch "スケッチ8" against normal blind 2 contours L27 L28 A14 L32 L26 | L27 L24 L32 A15 L11 L20 A14 L28 | A14 A10 L12 L32 | L28 A10 A14 | A14 L20 L28 | A10 L12 | L32 A12 A15 | A12 L20 | A12 L11 A15 picked at (-65.236512, -2.450134) picked at (-58.518516, -2.675024)
sketch "スケッチ10" plane through (0, 0, 0) normal (0, 0, 1) x (1, 0, 0)
  circle A0 centre (111.885049, -39.000002) radius 1.5
  circle A1 centre (61.312972, -56.131867) radius 13.85
  circle A2 centre (49.826136, -69.334238) radius 1.5
  circle A3 centre (49.826136, -69.334238) radius 3
  circle A4 centre (44.533686, -75.985551) radius 4
  circle A5 centre (61.312972, -56.131867) radius 14.5
  circle A6 centre (49.826136, -69.334238) radius 4
  circle A7 centre (44.533686, -75.985551) radius 7
  circle A8 centre (29.900285, -80.42716) radius 2
  circle A9 centre (29.900285, -80.42716) radius 8
  circle A10 centre (31.840112, -37) radius 7.5
  circle A11 centre (31.840112, -37) radius 34
  point P0 (0, 0)
  dimension "d101" = 6
  dimension "d102" = 8
  dimension "d103" = 29
  dimension "d104" = 1
  dimension "d105" = 3
  dimension "d106" = 16
  dimension "d107" = 68
  constraints: 12 centre point, 4 coincident, 2 tangent, 4 other
  measures "d101" diameter of A3
  measures "d102" diameter of A4
  measures "d103" diameter of A5
  measures "d104" radial gap between concentric circles of A3 A6
  measures "d105" radial gap between concentric circles of A4 A7
  measures "d106" diameter of A9
  measures "d107" diameter of A11
sketch "スケッチ11" plane through (0, 0, 0) normal (0, 0, 1) x (1, 0, 0)
  circle A0 centre (111.885049, -39.000002) radius 1.5
  circle A1 centre (61.312972, -56.131867) radius 13.85
  circle A2 centre (49.826136, -69.334238) radius 1.5
  circle A3 centre (49.826136, -69.334238) radius 3
  circle A4 centre (55.301358, -75.167071) radius 4
  circle A5 centre (61.312972, -56.131867) radius 14.5
  circle A6 centre (49.826136, -69.334238) radius 4
  circle A7 centre (55.301358, -75.167071) radius 7
  circle A8 centre (29.900285, -80.42716) radius 2
  circle A9 centre (29.900285, -80.42716) radius 8
  circle A10 centre (31.840112, -37) radius 7.5
  circle A11 centre (31.840112, -37) radius 34
  line L0 (47.462972, -56.050002) -> (47.462972, -31.350002)
  line L1 (49.444342, -3) -> (49.444342, -6)
  line L2 (49.444342, -6) -> (49.444342, -63.831309)
  line L3 (54.444342, -63.831309) -> (54.444342, -6)
  line L4 (54.444342, -6) -> (54.444342, -3)
  line L5 (51.301358, -31.350002) -> (51.301358, -56.050002)
  line L6 (51.301358, -56.050002) -> (51.301358, -80.750002)
  line L7 (51.301358, -80.750002) -> (-20.894321, -80.750002)
  point P0 (0, 0)
  dimension "d108" = 6
  dimension "d109" = 8
  dimension "d110" = 29
  dimension "d111" = 1
  dimension "d112" = 3
  dimension "d113" = 16
  dimension "d114" = 68
  dimension "d115" = 5
  constraints: 16 end point, 12 centre point, 5 vertical, 4 coincident, 3 collinear, 2 horizontal, 2 tangent, 5 other
  measures "d108" diameter of A3
  measures "d109" diameter of A4
  measures "d110" diameter of A5
  measures "d111" radial gap between concentric circles of A3 A6
  measures "d112" radial gap between concentric circles of A4 A7
  measures "d113" diameter of A9
  measures "d114" diameter of A11
  measures "d115" distance between parallel lines of L2 L3
sketch "スケッチ12" plane through (0, 0, 0) normal (0, 0, 1) x (1, 0, 0)
  circle A0 centre (111.885049, -39.000002) radius 1.5
  circle A1 centre (61.312972, -56.131867) radius 13.85
  circle A2 centre (49.826136, -69.334238) radius 1.5
  circle A3 centre (49.826136, -69.334238) radius 3
  circle A4 centre (61.312972, -56.131867) radius 14.5
  circle A5 centre (49.826136, -69.334238) radius 4
  circle A6 centre (29.900285, -80.42716) radius 2
  circle A7 centre (29.900285, -80.42716) radius 8
  circle A8 centre (31.840112, -37) radius 7.5
  circle A9 centre (31.840112, -37) radius 34
  line L0 (47.462972, -56.050002) -> (47.462972, -31.350002)
  line L1 (49.444342, -3) -> (49.444342, -6)
  line L2 (49.444342, -6) -> (49.444342, -63.831309)
  line L3 (54.301358, -63.831309) -> (54.301358, -6)
  line L4 (54.301358, -6) -> (54.301358, -3)
  line L5 (51.301358, -31.350002) -> (51.301358, -56.050002)
  line L6 (51.301358, -56.050002) -> (51.301358, -80.750002)
  line L7 (51.301358, -80.750002) -> (-20.894321, -80.750002)
  circle A10 centre (61.312972, -56.131867) radius 15.85
  line L8 (57.444342, -6) -> (57.444342, -3)
  arc A11 (59.444342, -3) -> (57.444342, -3) centre (58.444342, -3) ccw
  line L9 (59.444342, -3) -> (64.444342, -3)
  arc A12 (66.444342, -3) -> (64.444342, -3) centre (65.444342, -3) ccw
  line L10 (66.444342, -3) -> (66.444342, -6)
  arc A13 (64.444342, -6) -> (66.444342, -6) centre (65.444342, -6) ccw
  line L11 (64.444342, -6) -> (59.444342, -6)
  arc A14 (57.444342, -6) -> (59.444342, -6) centre (58.444342, -6) ccw
  arc A15 (89.889695, -3) -> (87.889695, -3) centre (88.889695, -3) ccw
  line L12 (89.889695, -3) -> (94.889695, -3)
  arc A16 (96.889695, -3) -> (94.889695, -3) centre (95.889695, -3) ccw
  line L13 (96.889695, -3) -> (96.889695, -6)
  arc A17 (94.889695, -6) -> (96.889695, -6) centre (95.889695, -6) ccw
  line L14 (94.889695, -6) -> (89.889695, -6)
  arc A18 (87.889695, -6) -> (89.889695, -6) centre (88.889695, -6) ccw
  line L15 (87.889695, -6) -> (87.889695, -3)
  circle A19 centre (111.885049, -39.000002) radius 1.5
  arc A20 (102.219392, -50.47062) -> (121.057661, -50.868582) centre (111.885049, -39.000002) ccw
  line L16 (121.057661, -50.868582) -> (127.651316, -45.772687)
  line L17 (127.651316, -45.772687) -> (126.808053, -37.482129)
  arc A21 (126.808053, -37.482129) -> (124.15135, -30.366471) centre (111.885049, -39.000002) ccw
  line L18 (124.15135, -30.366471) -> (104.889695, -3)
  line L19 (104.889695, -3) -> (101.889695, -3)
  arc A22 (99.889695, -3) -> (101.889695, -3) centre (100.889695, -3) ccw
  line L20 (99.889695, -3) -> (99.889695, 0)
  line L21 (99.889695, 0) -> (84.889695, 0)
  line L22 (84.889695, 0) -> (84.889695, -3)
  arc A23 (82.889695, -3) -> (84.889695, -3) centre (83.889695, -3) ccw
  line L23 (82.889695, -3) -> (71.444342, -3)
  arc A24 (69.444342, -3) -> (71.444342, -3) centre (70.444342, -3) ccw
  line L24 (69.444342, -3) -> (69.444342, 0)
  line L25 (69.444342, 0) -> (54.444342, 0)
  line L26 (54.444342, 0) -> (54.444342, -3)
  arc A25 (52.444342, -3) -> (54.444342, -3) centre (53.444342, -3) ccw
  line L27 (52.444342, -3) -> (49.444342, -3)
  line L28 (49.444342, -3) -> (49.444342, -6)
  line L29 (49.444342, -6) -> (102.219392, -50.47062)
  line L30 (54.301358, -63.831309) -> (54.301358, -70.007515)
  circle A26 centre (59.444342, -76.679981) radius 4
  point P0 (0, 0)
  dimension "d116" = 6
  dimension "d118" = 29
  dimension "d119" = 1
  dimension "d121" = 16
  dimension "d122" = 68
  dimension "d123" = 3
  dimension "d124" = 2
  dimension "d125" = 8
  constraints: 18 end point, 12 centre point, 6 vertical, 4 coincident, 3 collinear, 2 horizontal, 5 other
  measures "d116" diameter of A3
  measures "d118" diameter of A4
  measures "d119" radial gap between concentric circles of A3 A5
  measures "d121" diameter of A7
  measures "d122" diameter of A9
  measures "d123" distance between parallel lines of L3 L5
  measures "d124" radial gap between concentric circles of A1 A10
  measures "d125" diameter of A26
sketch "スケッチ13" plane through (0, 0, 0) normal (0, 0, 1) x (1, 0, 0)
  circle A0 centre (111.885049, -39.000002) radius 1.5
  circle A1 centre (61.312972, -56.131867) radius 13.85
  circle A2 centre (49.826136, -69.334238) radius 1.5
  circle A3 centre (49.826136, -69.334238) radius 3
  circle A4 centre (44.646096, -90.750002) radius 4
  circle A5 centre (61.312972, -56.131867) radius 14.5
  circle A6 centre (49.826136, -69.334238) radius 4
  circle A7 centre (44.646096, -90.750002) radius 7
  circle A8 centre (29.900285, -80.42716) radius 2
  circle A9 centre (29.900285, -80.42716) radius 8
  circle A10 centre (31.840112, -37) radius 7.5
  circle A11 centre (31.840112, -37) radius 34
  line L0 (47.462972, -56.050002) -> (47.462972, -31.350002)
  line L1 (49.444342, -3) -> (49.444342, -6)
  line L2 (49.444342, -6) -> (49.444342, -63.831309)
  line L3 (54.301358, -63.831309) -> (54.301358, -6)
  line L4 (54.301358, -6) -> (54.301358, -3)
  line L5 (51.301358, -31.350002) -> (51.301358, -56.050002)
  line L6 (51.301358, -56.050002) -> (51.301358, -80.750002)
  line L7 (51.301358, -80.750002) -> (-20.894321, -80.750002)
  circle A12 centre (61.312972, -56.131867) radius 15.85
  line L8 (-20.894321, -83.750002) -> (54.301358, -83.750002)
  line L9 (54.301358, -83.750002) -> (54.301358, -56.050002)
  line L10 (54.301358, -56.050002) -> (54.301358, -31.350002)
  arc A13 (104.885049, -31.858573) -> (119.12697, -45.895985) centre (111.885049, -39.000002) ccw
  line L11 (57.444342, -6) -> (57.444342, -3)
  arc A14 (59.444342, -3) -> (57.444342, -3) centre (58.444342, -3) ccw
  line L12 (59.444342, -3) -> (64.444342, -3)
  arc A15 (66.444342, -3) -> (64.444342, -3) centre (65.444342, -3) ccw
  line L13 (66.444342, -3) -> (66.444342, -6)
  arc A16 (64.444342, -6) -> (66.444342, -6) centre (65.444342, -6) ccw
  line L14 (64.444342, -6) -> (59.444342, -6)
  arc A17 (57.444342, -6) -> (59.444342, -6) centre (58.444342, -6) ccw
  arc A18 (89.889695, -3) -> (87.889695, -3) centre (88.889695, -3) ccw
  line L15 (89.889695, -3) -> (94.889695, -3)
  arc A19 (96.889695, -3) -> (94.889695, -3) centre (95.889695, -3) ccw
  line L16 (96.889695, -3) -> (96.889695, -6)
  arc A20 (94.889695, -6) -> (96.889695, -6) centre (95.889695, -6) ccw
  line L17 (94.889695, -6) -> (89.889695, -6)
  arc A21 (87.889695, -6) -> (89.889695, -6) centre (88.889695, -6) ccw
  line L18 (87.889695, -6) -> (87.889695, -3)
  circle A22 centre (111.885049, -39.000002) radius 1.5
  arc A23 (102.219392, -50.47062) -> (121.057661, -50.868582) centre (111.885049, -39.000002) ccw
  line L19 (121.057661, -50.868582) -> (127.651316, -45.772687)
  line L20 (127.651316, -45.772687) -> (126.808053, -37.482129)
  arc A24 (126.808053, -37.482129) -> (124.15135, -30.366471) centre (111.885049, -39.000002) ccw
  line L21 (124.15135, -30.366471) -> (104.889695, -3)
  line L22 (104.889695, -3) -> (101.889695, -3)
  arc A25 (99.889695, -3) -> (101.889695, -3) centre (100.889695, -3) ccw
  line L23 (99.889695, -3) -> (99.889695, 0)
  line L24 (99.889695, 0) -> (84.889695, 0)
  line L25 (84.889695, 0) -> (84.889695, -3)
  arc A26 (82.889695, -3) -> (84.889695, -3) centre (83.889695, -3) ccw
  line L26 (82.889695, -3) -> (71.444342, -3)
  arc A27 (69.444342, -3) -> (71.444342, -3) centre (70.444342, -3) ccw
  line L27 (69.444342, -3) -> (69.444342, 0)
  line L28 (69.444342, 0) -> (54.444342, 0)
  line L29 (54.444342, 0) -> (54.444342, -3)
  arc A28 (52.444342, -3) -> (54.444342, -3) centre (53.444342, -3) ccw
  line L30 (52.444342, -3) -> (49.444342, -3)
  line L31 (49.444342, -3) -> (49.444342, -6)
  line L32 (49.444342, -6) -> (102.219392, -50.47062)
  line L33 (48.373456, -96.6751) -> (119.87225, -51.69664)
  arc A29 (102.219392, -50.47062) -> (121.057661, -50.868582) centre (111.885049, -39.000002) ccw
  arc A30 (102.219392, -50.47062) -> (121.057661, -50.868582) centre (111.885049, -39.000002) ccw
  line L34 (-20.894321, -95.750002) -> (66.301358, -95.750002)
  line L35 (66.301358, -95.750002) -> (66.301358, -56.050002)
  line L36 (66.301358, -56.050002) -> (66.301358, -31.350002)
  point P0 (0, 0)
  point P1 (44.646096, -83.750002)
  point P2 (49.545076, -95.750002)
  point P3 (66.301358, -85.397016)
  point P4 (54.301358, -10.092739)
  dimension "d126" = 6
  dimension "d127" = 8
  dimension "d128" = 29
  dimension "d129" = 1
  dimension "d130" = 3
  dimension "d131" = 16
  dimension "d132" = 68
  dimension "d133" = 3
  dimension "d134" = 2
  dimension "d135" = 3
  dimension "d136" = 18
  dimension "d137" = 12
  constraints: 30 end point, 12 centre point, 4 coincident, 3 collinear, 3 horizontal, 2 vertical, 1 point on circle, 1 tangent, 13 other
  measures "d126" diameter of A3
  measures "d127" diameter of A4
  measures "d128" diameter of A5
  measures "d129" radial gap between concentric circles of A3 A6
  measures "d131" diameter of A9
  measures "d132" diameter of A11
  measures "d133" distance between parallel lines of L3 L5
  measures "d134" radial gap between concentric circles of A1 A12
  measures "d135" distance between parallel lines of L7 L8
  measures "d136" distance of A8.centre A4.centre
  measures "d137" distance between parallel lines of L8 L34
sketch "スケッチ14" plane through (0, 0, 0) normal (0, 0, 1) x (1, 0, 0)
  line L0 (57.444342, -6) -> (57.444342, -3)
  arc A0 (59.444342, -3) -> (57.444342, -3) centre (58.444342, -3) ccw
  line L1 (59.444342, -3) -> (64.444342, -3)
  arc A1 (66.444342, -3) -> (64.444342, -3) centre (65.444342, -3) ccw
  line L2 (66.444342, -3) -> (66.444342, -6)
  arc A2 (64.444342, -6) -> (66.444342, -6) centre (65.444342, -6) ccw
  line L3 (64.444342, -6) -> (59.444342, -6)
  arc A3 (57.444342, -6) -> (59.444342, -6) centre (58.444342, -6) ccw
  arc A4 (89.889695, -3) -> (87.889695, -3) centre (88.889695, -3) ccw
  line L4 (89.889695, -3) -> (94.889695, -3)
  arc A5 (96.889695, -3) -> (94.889695, -3) centre (95.889695, -3) ccw
  line L5 (96.889695, -3) -> (96.889695, -6)
  arc A6 (94.889695, -6) -> (96.889695, -6) centre (95.889695, -6) ccw
  line L6 (94.889695, -6) -> (89.889695, -6)
  arc A7 (87.889695, -6) -> (89.889695, -6) centre (88.889695, -6) ccw
  line L7 (87.889695, -6) -> (87.889695, -3)
  circle A8 centre (111.885049, -39.000002) radius 1.5
  arc A9 (102.219392, -50.47062) -> (121.057661, -50.868582) centre (111.885049, -39.000002) ccw
  line L8 (121.057661, -50.868582) -> (127.651316, -45.772687)
  line L9 (127.651316, -45.772687) -> (126.808053, -37.482129)
  arc A10 (126.808053, -37.482129) -> (124.15135, -30.366471) centre (111.885049, -39.000002) ccw
  line L10 (124.15135, -30.366471) -> (104.889695, -3)
  line L11 (104.889695, -3) -> (101.889695, -3)
  arc A11 (99.889695, -3) -> (101.889695, -3) centre (100.889695, -3) ccw
  line L12 (99.889695, -3) -> (99.889695, 0)
  line L13 (99.889695, 0) -> (84.889695, 0)
  line L14 (84.889695, 0) -> (84.889695, -3)
  arc A12 (82.889695, -3) -> (84.889695, -3) centre (83.889695, -3) ccw
  line L15 (82.889695, -3) -> (71.444342, -3)
  arc A13 (69.444342, -3) -> (71.444342, -3) centre (70.444342, -3) ccw
  line L16 (69.444342, -3) -> (69.444342, 0)
  line L17 (69.444342, 0) -> (54.444342, 0)
  line L18 (54.444342, 0) -> (54.444342, -3)
  arc A14 (52.444342, -3) -> (54.444342, -3) centre (53.444342, -3) ccw
  line L19 (52.444342, -3) -> (49.444342, -3)
  line L20 (49.444342, -3) -> (49.444342, -6)
  line L21 (49.444342, -6) -> (102.219392, -50.47062)
  point P0 (0, 0)